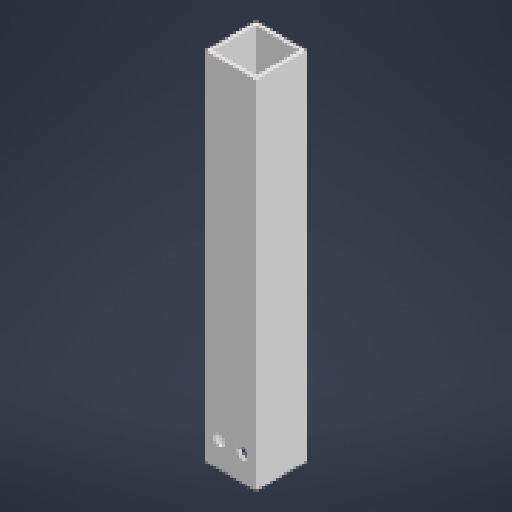
# Autodesk Inventor part: 1
Saved by Autodesk Inventor 2024 (Build 280153000, 153)
## iProperties
Created: 2023-04-17
Part Number: 1
Material: Алюминий 6061
Document SubType Name: Modeling
Designer: user
Mass: 41.7544 g
Surface Area: 209.169 cm^2
Volume: 15.4646 cm^3
Density: 2.7 g/cm^3
Appearance: Алюминий — плоский
Author: user
Autodesk Inventor part; units mm, degrees
ref_plane "YZ Plane" through (0, 0, 0) normal (1, 0, 0) x (0, 1, 0)
ref_plane "XZ Plane" through (0, 0, 0) normal (0, 1, 0) x (-1, 0, 0)
ref_plane "XY Plane" through (0, 0, 0) normal (0, 0, 1) x (1, 0, 0)
sketch "Эскиз1" plane through (0, 0, 0) normal (0, 0, 1) x (1, 0, 0)
  line L0 (0, 0) -> (20, 0)
  line L1 (20, 0) -> (20, 20)
  line L2 (20, 20) -> (0, 20)
  line L3 (0, 20) -> (0, 0)
  line L4 (1.5, 1.5) -> (18.5, 1.5)
  line L5 (18.5, 1.5) -> (18.5, 18.5)
  line L6 (18.5, 18.5) -> (1.5, 18.5)
  line L7 (1.5, 18.5) -> (1.5, 1.5)
  point P0 (10, 18.5)
  point P1 (10, 20)
  point P2 (18.5, 10)
  point P3 (20, 10)
  dimension "d0" = 20
  dimension "d1" = 1.5
  constraints: 16 end point, 4 midpoint, 4 parallel, 4 perpendicular, 2 horizontal, 1 horizontal alignment, 1 vertical alignment
  measures "d0" distance of L0.end L1.end
  measures "d1" horizontal distance of L1.end L5.end
extrude "Выдавливание1" add sketch "Эскиз1" along normal blind 140
sketch "Эскиз2" plane through (0, 20, 0) normal (0, 1, 0) x (1, 0, 0)
  circle A0 centre (6, -10) radius 2
  circle A1 centre (14, -10) radius 2
  line L0 (14, -10) -> (6, -10) construction
  line L1 (20, 0) -> (0, 0) construction
  point P0 (10, -10)
  point P1 (10, 0)
  dimension "d4" = 10
  dimension "d5" = 4
  dimension "d8" = 8
  constraints: 2 centre point, 2 end point, 2 midpoint, 1 equal radius, 1 horizontal, 1 horizontal alignment, 1 vertical alignment
  measures "d4" vertical distance of L1.end L0.end
  measures "d5" diameter of A0
  measures "d8" distance of L0.start L0.end
extrude "Выдавливание2" cut sketch "Эскиз2" against normal through all
